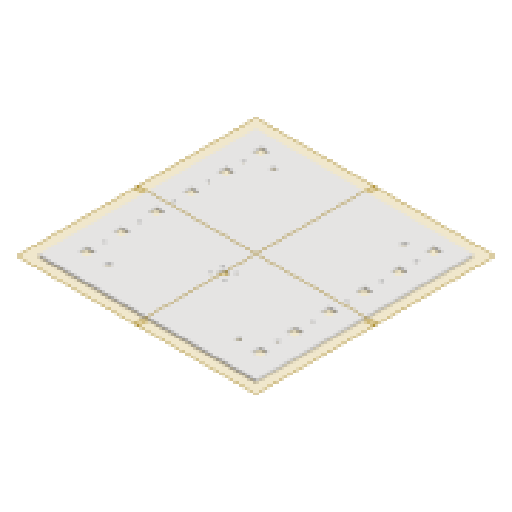
# Autodesk Inventor part: Основание подъёмника
Saved by Autodesk Inventor 2023.2 (Build 272271030, 271C)
## iProperties
Created: 2025-03-19
Part Number: Основание подъёмника
Material: Типовые
Document SubType Name: Modeling
Designer: Коноваленко
Density: 1 g/cm^3
Appearance: По умолчанию
Author: Коноваленко
Autodesk Inventor part; units mm, degrees
sketch "Эскиз1" plane through (0, 0, 0) normal (0, 1, 0) x (-1, 0, 0)
  line L0 (125, 125) -> (-125, 125)
  line L1 (-125, 125) -> (-125, -125)
  line L2 (-125, -125) -> (125, -125)
  line L3 (125, -125) -> (125, 125)
  line L4 (125, 125) -> (-125, -125) construction
  line L5 (-125, 125) -> (125, -125) construction
  point P0 (0, 0)
  dimension "d0" = 250
  dimension "d1" = 250
  constraints: 12 end point, 2 midpoint, 2 parallel, 1 horizontal, 1 perpendicular
  measures "d0" distance of L0.end L1.end
  measures "d1" distance of L1.end L2.end
extrude "Выдавливание1" add sketch "Эскиз1" along normal mid plane 4
sketch "Эскиз2" plane through (0, -2, 0) normal (0, -1, 0) x (1, 0, 0)
  line L0 (104.5, -110) -> (104.5, -100) projected
  line L1 (104.5, -100) -> (94.5, -100) projected
  line L2 (94.5, -100) -> (94.5, -110) projected
  line L3 (94.5, -110) -> (104.5, -110) projected
  circle A0 centre (99.5, -85) radius 2 projected
  line L4 (104.5, -70) -> (104.5, -60) projected
  line L5 (104.5, -60) -> (94.5, -60) projected
  line L6 (94.5, -60) -> (94.5, -70) projected
  line L7 (94.5, -70) -> (104.5, -70) projected
  circle A1 centre (99.5, -45) radius 2 projected
  line L8 (104.5, -30) -> (104.5, -20) projected
  line L9 (104.5, -20) -> (94.5, -20) projected
  line L10 (94.5, -20) -> (94.5, -30) projected
  line L11 (94.5, -30) -> (104.5, -30) projected
  circle A2 centre (99.5, -5) radius 2 projected
  line L12 (104.5, 10) -> (104.5, 20) projected
  line L13 (104.5, 20) -> (94.5, 20) projected
  line L14 (94.5, 20) -> (94.5, 10) projected
  line L15 (94.5, 10) -> (104.5, 10) projected
  circle A3 centre (99.5, 35) radius 2 projected
  line L16 (94.5, 55) -> (94.5, 50) projected
  line L17 (94.5, 50) -> (104.5, 50) projected
  line L18 (104.5, 50) -> (104.5, 55) projected
  line L19 (104.5, 55) -> (104.5, 60) projected
  line L20 (104.5, 60) -> (94.5, 60) projected
  line L21 (94.5, 60) -> (94.5, 55) projected
  line L22 (104.5, 90) -> (104.5, 100) projected
  line L23 (104.5, 100) -> (94.5, 100) projected
  line L24 (94.5, 100) -> (94.5, 90) projected
  line L25 (94.5, 90) -> (104.5, 90) projected
  line L26 (-104.5, 90) -> (-104.5, 100) projected
  line L27 (-94.5, 90) -> (-104.5, 90) projected
  line L28 (-94.5, 100) -> (-94.5, 90) projected
  line L29 (-104.5, 100) -> (-94.5, 100) projected
  line L30 (-104.5, 50) -> (-104.5, 55) projected
  line L31 (-94.5, 50) -> (-104.5, 50) projected
  line L32 (-94.5, 55) -> (-94.5, 50) projected
  line L33 (-94.5, 60) -> (-94.5, 55) projected
  line L34 (-104.5, 60) -> (-94.5, 60) projected
  line L35 (-104.5, 55) -> (-104.5, 60) projected
  line L36 (-104.5, 10) -> (-104.5, 20) projected
  line L37 (-94.5, 10) -> (-104.5, 10) projected
  line L38 (-94.5, 20) -> (-94.5, 10) projected
  line L39 (-104.5, 20) -> (-94.5, 20) projected
  line L40 (-104.5, -30) -> (-104.5, -20) projected
  line L41 (-94.5, -30) -> (-104.5, -30) projected
  line L42 (-94.5, -20) -> (-94.5, -30) projected
  line L43 (-104.5, -20) -> (-94.5, -20) projected
  line L44 (-104.5, -70) -> (-104.5, -60) projected
  line L45 (-94.5, -70) -> (-104.5, -70) projected
  line L46 (-94.5, -60) -> (-94.5, -70) projected
  line L47 (-104.5, -60) -> (-94.5, -60) projected
  line L48 (-104.5, -110) -> (-104.5, -100) projected
  line L49 (-94.5, -110) -> (-104.5, -110) projected
  line L50 (-94.5, -100) -> (-94.5, -110) projected
  line L51 (-104.5, -100) -> (-94.5, -100) projected
  circle A4 centre (-99.5, -85) radius 2 projected
  circle A5 centre (-99.5, -45) radius 2 projected
  circle A6 centre (-99.5, -5) radius 2 projected
  circle A7 centre (-99.5, 35) radius 2 projected
  circle A8 centre (-99.5, 75) radius 2 projected
  circle A9 centre (99.5, 75) radius 2 projected
extrude "Выдавливание2" cut sketch "Эскиз2" against normal up to surface (4 mm away)
sketch "Эскиз3" plane through (0, -2, 0) normal (0, -1, 0) x (1, 0, 0)
  circle A0 centre (75, -95) radius 3.15
  line L0 (125, -125) -> (125, 125) projected
  line L1 (-125, -125) -> (125, -125) projected
  line L2 (0, -76.118) -> (0, 76.118) construction
  line L3 (24.9561, 0) -> (-24.9561, 0) construction
  circle A1 centre (-75, -95) radius 3.15
  line L4 (-24.9561, 0) -> (24.9561, 0) construction
  circle A2 centre (75, 95) radius 3.15
  circle A3 centre (-75, 95) radius 3.15
  point P0 (0, 0)
  point P1 (0, 0)
  dimension "d10" = 6.3
  dimension "d14" = 50
  dimension "d15" = 30
  constraints: 6 end point, 5 symmetric about line, 4 centre point, 2 midpoint, 1 coincident, 1 horizontal, 1 vertical, 3 other
  measures "d10" diameter of A0
  measures "d14" distance from line of L0 A0.centre
  measures "d15" distance from line of L1 A0.centre
extrude "Выдавливание3" cut sketch "Эскиз3" against normal up to surface (4 mm away)
sketch "Эскиз4" plane through (0, -2, 0) normal (0, -1, 0) x (1, 0, 0)
  circle A0 centre (-8, 44.7403) radius 1.85
  circle A1 centre (-8, 30.7403) radius 1.85
  circle A2 centre (0, 37.7403) radius 5
  circle A3 centre (8, 44.7403) radius 1.85
  circle A4 centre (8, 30.7403) radius 1.85
  point P0 (0, 0)
  constraints: 5 centre point, 10 other
extrude "Выдавливание4" cut sketch "Эскиз4" against normal up to surface (4 mm away)
